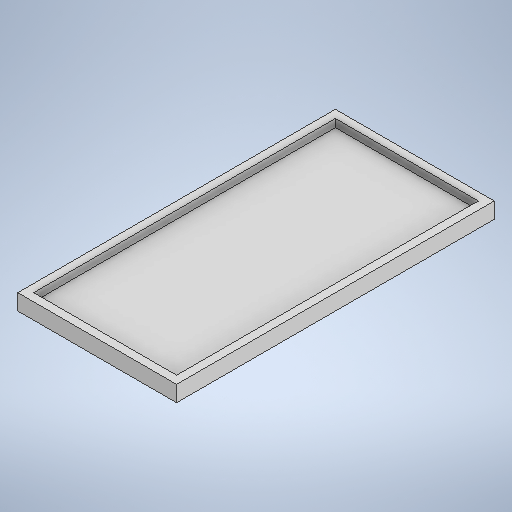
# Autodesk Inventor part: Potting Tray
Saved by Autodesk Inventor 2025 (Build 290162000, 162)
## iProperties
Created: 2024-06-19
Part Number: Potting Tray
Material: Generic
Document SubType Name: Modeling
Designer: User
Density: 1 g/cm^3
Appearance: Default
Author: User
Autodesk Inventor part; units mm, degrees
ref_plane "YZ Plane" through (0, 0, 0) normal (1, 0, 0) x (0, 1, 0)
ref_plane "XZ Plane" through (0, 0, 0) normal (0, 1, 0) x (-1, 0, 0)
ref_plane "XY Plane" through (0, 0, 0) normal (0, 0, 1) x (1, 0, 0)
sketch "Sketch1" plane through (0, 0, 0) normal (0, 1, 0) x (-1, 0, 0)
  line L0 (-127, 254) -> (127, 254)
  line L1 (127, 254) -> (127, -254)
  line L2 (127, -254) -> (-127, -254)
  line L3 (-127, -254) -> (-127, 254)
  line L4 (-127, 254) -> (127, -254) construction
  line L5 (127, 254) -> (-127, -254) construction
  line L6 (-114.3, 241.3) -> (114.3, 241.3)
  line L7 (114.3, 241.3) -> (114.3, -241.3)
  line L8 (114.3, -241.3) -> (-114.3, -241.3)
  line L9 (-114.3, -241.3) -> (-114.3, 241.3)
  line L10 (-114.3, 241.3) -> (114.3, -241.3) construction
  line L11 (114.3, 241.3) -> (-114.3, -241.3) construction
  point P0 (0, 0)
  dimension "d0" = 508
  dimension "d1" = 254
  dimension "d2" = 482.6
  dimension "d3" = 228.6
  constraints: 24 end point, 4 midpoint, 4 parallel, 2 horizontal, 2 perpendicular
  measures "d0" distance of L0.end L1.end
  measures "d1" distance of L1.end L2.end
  measures "d2" distance of L6.end L7.end
  measures "d3" distance of L7.end L8.end
extrude "Extrusion1" add sketch "Sketch1" along normal blind 12.7 contours L6 L7 L8 L9
extrude "Extrusion2" add sketch "Sketch1" along normal blind 25.4
body "Solid1"
